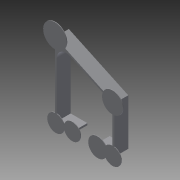
# Autodesk Inventor part: Stand
Saved by Autodesk Inventor 2014 SP1 (Build 180222100, 222)
## iProperties
Created: 2014-08-07
Part Number: Stand
Material: Generic
Document SubType Name: Modeling
Designer: Erin
Density: 1 g/cm^3
Appearance: Default
Author: Erin
Autodesk Inventor part; units mm, degrees
ref_plane "YZ Plane" through (0, 0, 0) normal (1, 0, 0) x (0, 1, 0)
ref_plane "XZ Plane" through (0, 0, 0) normal (0, 1, 0) x (-1, 0, 0)
ref_plane "XY Plane" through (0, 0, 0) normal (0, 0, 1) x (1, 0, 0)
sketch "Sketch1" plane through (0, 0, 0) normal (0, 1, 0) x (-1, 0, 0)
  line L0 (-16.6929, 0.141) -> (47.3831, 30.0201)
  line L1 (-16.6929, 0.141) -> (62.5092, 0.141) construction
  line L2 (-16.6929, 0.141) -> (-16.6929, -49.859)
  line L3 (47.3831, 30.0201) -> (47.3831, -49.859)
  line L4 (-16.6929, -49.859) -> (3.3071, -49.859)
  line L5 (47.3831, -49.859) -> (27.3831, -49.859)
  line L6 (27.3831, -47.859) -> (45.3831, -47.859)
  line L7 (45.3831, -47.859) -> (45.3831, 26.8807)
  line L8 (45.3831, 26.8807) -> (-14.6929, -1.1332)
  line L9 (-14.6929, -1.1332) -> (-14.6929, -47.859)
  line L10 (-14.6929, -47.859) -> (3.3071, -47.859)
  line L11 (3.3071, -49.859) -> (3.3071, -47.859)
  line L12 (27.3831, -49.859) -> (27.3831, -47.859)
  point P0 (0, 0)
  dimension "d0" = 70.7
  dimension "d1" = 25
  dimension "d2" = 50
  dimension "d3" = 20
  dimension "d5" = 20
  dimension "d6" = 2
  dimension "d7" = 2
  constraints: 26 end point, 3 perpendicular, 2 collinear, 2 parallel, 1 horizontal
  measures "d0" distance of L0.start L0.end
  measures "d1" angle of L1 L0
  measures "d2" distance of L0.start L2.end
  measures "d3" distance of L2.end L4.end
  measures "d5" distance of L3.end L5.end
  measures "d6" distance between parallel lines of L2 L9
  measures "d7" distance between parallel lines of L3 L7
extrude "Extrusion1" add sketch "Sketch1" along normal blind 15
fillet "Fillet1" radius 10 2 edges at (-45.3831, 7.5, 26.8807) (14.6929, 7.5, -1.1332)
sketch "Sketch2" plane through (0, 0, 0) normal (0, -1, 0) x (1, 0, 0)
  line L0 (-47.3831, -49.859) -> (-27.3831, -49.859) projected
  line L1 (-3.3071, -49.859) -> (16.6929, -49.859) projected
  circle A0 centre (-47.3831, 31.2222) radius 12.7105
  circle A1 centre (14.6929, 0) radius 11.2925
  circle A2 centre (-46.4362, -49.859) radius 9.2192
  circle A3 centre (-28.7772, -48.859) radius 9.0347
  circle A4 centre (-1.3494, -49.859) radius 10.1488
  circle A5 centre (14.6929, -49.859) radius 9.416
  point P0 (0, 0)
  constraints: 6 centre point, 3 point on line
extrude "Extrusion2" add sketch "Sketch2" against normal blind 0.6
body "Solid1"
